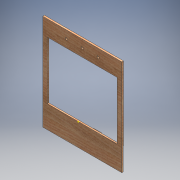
# Autodesk Inventor part: Base
Saved by Autodesk Inventor 2016 (Build 200138000, 138)
## iProperties
Created: 2016-04-01
Part Number: Base
Material: Wood (Birch)
Document SubType Name: Modeling
Designer: mkepler
Density: 0.55 g/cm^3
Appearance: Birch - Natural Polished
Mass: 193.765 g
Surface Area: 997.803 cm^2
Volume: 352.3 cm^3
Author: mkepler
Autodesk Inventor part; units mm, degrees
ref_plane "YZ Plane" through (0, 0, 0) normal (1, 0, 0) x (0, 1, 0)
ref_plane "XZ Plane" through (0, 0, 0) normal (0, 1, 0) x (-1, 0, 0)
ref_plane "XY Plane" through (0, 0, 0) normal (0, 0, 1) x (1, 0, 0)
sketch "Sketch1" plane through (0, 0, 0) normal (0, 1, 0) x (-1, 0, 0)
  line L0 (0, 0) -> (350, 0)
  line L1 (350, 0) -> (350, -100)
  line L2 (350, -100) -> (0, -100)
  line L3 (0, -100) -> (0, 0)
  dimension "d0" = 350
  dimension "d1" = 100
  constraints: 8 end point, 2 parallel, 1 horizontal, 1 perpendicular
  measures "d0" distance of L1.end L2.end
  measures "d1" distance of L0.end L1.end
extrude "Extrusion1" add sketch "Sketch1" along normal blind 6.35
sketch "Sketch2" plane through (0, 6.35, 0) normal (0, 1, 0) x (1, 0, 0)
  line L0 (0, 100) -> (-350, 100) projected
  line L1 (-192.5, 100) -> (-157.5, 100)
  line L2 (-157.5, 100) -> (-157.5, 60)
  line L3 (-157.5, 60) -> (-192.5, 60)
  line L4 (-192.5, 60) -> (-192.5, 100)
  line L5 (0, 0) -> (0, 100) projected
  dimension "d10" = 35
  dimension "d11" = 40
  dimension "d12" = 157.5
  constraints: 8 end point, 2 parallel, 1 horizontal, 1 perpendicular, 1 point on line
  measures "d10" distance of L2.end L3.end
  measures "d11" distance of L1.end L2.end
  measures "d12" distance between parallel lines of L5 L2
extrude "Extrusion2" add sketch "Sketch2" along normal blind 62
sketch "Sketch3" plane through (0, 68.35, 0) normal (0, 1, 0) x (1, 0, 0)
  circle A0 centre (-175, 94) radius 2.125
  line L0 (-157.5, 100) -> (-192.5, 100) projected
  circle A1 centre (-169, 94) radius 2.125
  circle A2 centre (-181, 94) radius 2.125
  point P0 (0, 0)
  dimension "d15" = 4.25
  dimension "d16" = 6
  dimension "d17" = 4.25
  dimension "d18" = 6
  dimension "d19" = 4.25
  dimension "d20" = 6
  constraints: 3 centre point
  measures "d15" diameter of A0
  measures "d16" distance from line of L0 A0.centre
  measures "d17" diameter of A1
  measures "d18" distance of A0.centre A1.centre
  measures "d19" diameter of A2
  measures "d20" distance of A0.centre A2.centre
hole "Hole1" at (-181, 68.35, -94) at (-175, 68.35, -94) at (-169, 68.35, -94) direction (0, -1, 0) diameter 4.25 depth 8 tip angle 118
sketch "Sketch4" plane through (-192.5, 6.35, -100) normal (-1, 0, 0) x (0, 0, 1)
  point P0 (100, -6.35)
sketch "Sketch5" plane through (-192.5, 6.35, -100) normal (-1, 0, 0) x (0, 0, 1)
  line L0 (0, 0) -> (0, 62) projected
  line L1 (0, 42) -> (40, 42)
  line L2 (40, 0) -> (40, 62) projected
  line L3 (0, 62) -> (40, 62) projected
  circle A0 centre (6, 48) radius 1.5
  circle A1 centre (34, 48) radius 1.5
  point P0 (100, -6.35)
  dimension "d28" = 20
  dimension "d29" = 3
  dimension "d30" = 3
  dimension "d31" = 6
  dimension "d32" = 6
  dimension "d33" = 6
  dimension "d34" = 6
  constraints: 2 centre point, 2 end point, 2 point on line, 1 horizontal
  measures "d28" distance between parallel lines of L1 L3
  measures "d29" diameter of A0
  measures "d30" diameter of A1
  measures "d31" distance from line of L2 A1.centre
  measures "d32" distance from line of L0 A0.centre
  measures "d33" distance from line of L1 A1.centre
  measures "d34" distance from line of L1 A0.centre
hole "Hole2" at (-192.5, 54.35, -66) at (-192.5, 54.35, -94) direction (1, 0, 0) diameter 3 depth 2 tip angle 118
sketch "Sketch6" plane through (-192.5, 6.35, -60) normal (0, 0, 1) x (1, 0, 0)
  line L0 (0, 42) -> (35, 42)
  line L1 (0, 62) -> (35, 62) projected
  circle A0 centre (6, 48) radius 1.5
  line L2 (0, 0) -> (0, 62) projected
  circle A1 centre (29, 48) radius 1.5
  line L3 (35, 0) -> (35, 62) projected
  point P0 (192.5, -6.35)
  dimension "d42" = 20
  dimension "d43" = 3
  dimension "d44" = 6
  dimension "d45" = 6
  dimension "d46" = 3
  dimension "d47" = 6
  dimension "d48" = 6
  constraints: 2 centre point, 2 end point, 1 horizontal
  measures "d42" distance between parallel lines of L0 L1
  measures "d43" diameter of A0
  measures "d44" distance from line of L2 A0.centre
  measures "d45" distance from line of L0 A0.centre
  measures "d46" diameter of A1
  measures "d47" distance from line of L0 A1.centre
  measures "d48" distance from line of A1.centre L3
hole "Hole3" at (-186.5, 54.35, -60) at (-163.5, 54.35, -60) direction (0, 0, -1) diameter 3 depth 2 tip angle 118
sketch "Sketch7" plane through (-157.5, 6.35, -60) normal (1, 0, 0) x (0, 0, -1)
  circle A0 centre (6, 48) radius 1.5 projected
  circle A1 centre (6, 48) radius 1.5
  circle A2 centre (34, 48) radius 1.5 projected
  circle A3 centre (34, 48) radius 1.5
  point P0 (-60, -6.35)
  dimension "d56" = 3
  dimension "d57" = 3
  constraints: 2 centre point, 2 coincident
  measures "d56" diameter of A1
  measures "d57" diameter of A3
hole "Hole4" at (-157.5, 54.35, -66) at (-157.5, 54.35, -94) direction (-1, 0, 0) diameter 3 depth 2 tip angle 118
sketch "Sketch8" plane through (0, 0, 0) normal (0, -1, 0) x (1, 0, 0)
  line L0 (-350, -100) -> (0, -100) projected
  line L1 (-350, -100) -> (-330, -100)
  line L2 (-330, 0) -> (-330, 255)
  line L3 (-330, 325) -> (-350, 325)
  line L4 (-350, 325) -> (-350, 0)
  line L5 (-350, 325) -> (0, 325)
  line L6 (0, 0) -> (0, -100) projected
  line L7 (0, 325) -> (0, 0)
  line L8 (0, -100) -> (-20, -100)
  line L9 (0, -100) -> (-157.5, -100) projected
  line L10 (-20, 0) -> (-20, 255)
  line L11 (-20, 325) -> (50, 325) construction
  line L12 (-20, 255) -> (-330, 255)
  line L13 (-350, 0) -> (0, 0) projected
  line L14 (-350, 0) -> (-330, 0)
  line L15 (-20, 0) -> (0, 0)
  dimension "d65" = 20
  dimension "d66" = 425
  constraints: 24 end point, 8 point on line, 6 perpendicular, 1 horizontal
  measures "d65" distance of L0.start L1.end
  measures "d66" distance of L1.end L3.start
extrude "Extrusion3" add sketch "Sketch8" against normal blind 7.5 contours L13 L4 L3 L5 L7 L10 L12 L2
sketch "Sketch9" plane through (0, 7.5, 0) normal (0, 1, 0) x (1, 0, 0)
  line L0 (-20, -255) -> (-330, -255) projected
  line L1 (-175, -255) -> (-175, -325)
  line L2 (-350, -325) -> (0, -325) projected
  line L3 (-175, -290) -> (-168, -290)
  line L4 (0, 100) -> (0, -325) projected
  line L5 (-168, -290) -> (-134.9357, -290)
  circle A0 centre (-175, -290) radius 5
  circle A1 centre (-105, -290) radius 5
  circle A2 centre (-245, -290) radius 5
  point P0 (0, 0)
  dimension "d73" = 7
  dimension "d74" = 10
  dimension "d75" = 10
  dimension "d76" = 10
  dimension "d77" = 70
  dimension "d78" = 70
  constraints: 6 end point, 3 centre point, 3 midpoint, 1 coincident, 1 perpendicular, 1 point on line
  measures "d73" distance of L3.start L3.end
  measures "d74" diameter of A0
  measures "d75" diameter of A1
  measures "d76" diameter of A2
  measures "d77" distance of L3.start A1.centre
  measures "d78" distance of A2.centre L3.start
hole "Hole5" at (-105, 7.5, 290) at (-175, 7.5, 290) at (-245, 7.5, 290) direction (0, -1, 0) diameter 10 depth 8 tip angle 118
body "Solid1"
